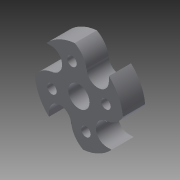
# Autodesk Inventor part: ratchet
Saved by Autodesk Inventor 2013 (Build 170138000, 138)
## iProperties
Created: 2014-01-04
Part Number: ratchet
Material: Generic
Document SubType Name: Modeling
Designer: kahohbein
Density: 1 g/cm^3
Author: kahohbein
Autodesk Inventor part; units mm, degrees
ref_plane "YZ Plane" through (0, 0, 0) normal (1, 0, 0) x (0, 1, 0)
ref_plane "XZ Plane" through (0, 0, 0) normal (0, 1, 0) x (-1, 0, 0)
ref_plane "XY Plane" through (0, 0, 0) normal (0, 0, 1) x (1, 0, 0)
sketch "Sketch1" plane through (0, 0, 0) normal (0, 0, 1) x (1, 0, 0)
  line L0 (-9.3495, 8.5951) -> (-8.0128, 8.5951)
  arc A0 (-8.0128, 2.2451) -> (-8.0128, 8.5951) centre (-8.0128, 5.4201) ccw
  line L1 (-8.0128, 2.2451) -> (-6.9824, 2.2451)
  arc A1 (-6.9824, 2.2451) -> (-12.641, -1.2233) centre (-6.9824, -4.1049) ccw
  line L2 (-8.5951, -9.3495) -> (-8.5951, -8.0128)
  arc A2 (-2.2451, -8.0128) -> (-8.5951, -8.0128) centre (-5.4201, -8.0128) ccw
  line L3 (-2.2451, -8.0128) -> (-2.2451, -6.9824)
  arc A3 (-2.2451, -6.9824) -> (1.2233, -12.641) centre (4.1049, -6.9824) ccw
  line L4 (9.3495, -8.5951) -> (8.0128, -8.5951)
  arc A4 (8.0128, -2.2451) -> (8.0128, -8.5951) centre (8.0128, -5.4201) ccw
  line L5 (8.0128, -2.2451) -> (6.9824, -2.2451)
  arc A5 (6.9824, -2.2451) -> (12.641, 1.2233) centre (6.9824, 4.1049) ccw
  line L6 (8.5951, 9.3495) -> (8.5951, 8.0128)
  arc A6 (2.2451, 8.0128) -> (8.5951, 8.0128) centre (5.4201, 8.0128) ccw
  line L7 (2.2451, 8.0128) -> (2.2451, 6.9824)
  arc A7 (2.2451, 6.9824) -> (-1.2233, 12.641) centre (-4.1049, 6.9824) ccw
  arc A8 (-1.2233, 12.641) -> (-9.3495, 8.5951) centre (0, 0) ccw
  arc A9 (12.641, 1.2233) -> (8.5951, 9.3495) centre (0, 0) ccw
  arc A10 (-12.641, -1.2233) -> (-8.5951, -9.3495) centre (0, 0) ccw
  arc A11 (1.2233, -12.641) -> (9.3495, -8.5951) centre (0, 0) ccw
  point P0 (-12.4977, 2.2451)
  point P1 (-2.2451, -12.4977)
  point P2 (12.4977, -2.2451)
  point P3 (2.2451, 12.4977)
  dimension "d1" = 6.35
  dimension "d2" = 6.35
  dimension "d5" = 360
  constraints: 24 point on circle, 16 end point, 12 centre point, 4 point on line, 3 tangent, 1 coincident, 1 horizontal, 1 parallel, 53 other
  measures "d1" diameter of A0
  measures "d2" radius of A1
extrude "Extrusion1" add sketch "Sketch1" along normal blind 6.35
sketch "Sketch2" plane through (0, 0, 6.35) normal (0, 0, 1) x (1, 0, 0)
  arc A0 (-1.2233, 12.641) -> (-9.3495, 8.5951) centre (0, 0) ccw projected
  circle A1 centre (0, 0) radius 3.048
  dimension "d9" = 6.096
  constraints: 1 centre point, 1 coincident
  measures "d9" diameter of A1
extrude "Extrusion2" cut sketch "Sketch2" against normal blind 6.35
sketch "Sketch3" plane through (0, 0, 6.35) normal (0, 0, 1) x (1, 0, 0)
  arc A0 (-6.9824, 2.2451) -> (-12.641, -1.2233) centre (-6.9824, -4.1049) ccw projected
  arc A1 (-2.2451, -6.9824) -> (1.2233, -12.641) centre (4.1049, -6.9824) ccw projected
  arc A2 (6.9824, -2.2451) -> (12.641, 1.2233) centre (6.9824, 4.1049) ccw projected
  arc A3 (2.2451, 6.9824) -> (-1.2233, 12.641) centre (-4.1049, 6.9824) ccw projected
  circle A4 centre (-7.7473, -1.9949) radius 1.3525
  circle A5 centre (-1.9949, 7.7473) radius 1.3525
  circle A6 centre (7.7473, 1.9949) radius 1.3525
  circle A7 centre (1.9949, -7.7473) radius 1.3525
  line L0 (7.7473, 1.9949) -> (6.9824, 4.1049)
  line L1 (-1.9949, 7.7473) -> (-4.1049, 6.9824)
  line L2 (-7.7473, -1.9949) -> (-6.9824, -4.1049)
  line L3 (1.9949, -7.7473) -> (4.1049, -6.9824)
  constraints: 8 end point, 6 perpendicular, 4 centre point
extrude "Extrusion3" cut sketch "Sketch3" against normal blind 6.35
body "Solid1"
